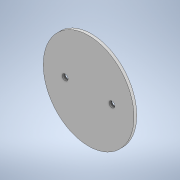
# Autodesk Inventor part: Plato da Valvula
Saved by Autodesk Inventor 2022 (Build 260153000, 153)
## iProperties
Created: 2022-06-22
Part Number: Plato da Valvula
Material: Genérico
Document SubType Name: Modeling
Designer: robofei
Density: 1 g/cm^3
Appearance: Padrão
Author: robofei
Autodesk Inventor part; units mm, degrees
ref_plane "YZ Plane" through (0, 0, 0) normal (1, 0, 0) x (0, 1, 0)
ref_plane "XZ Plane" through (0, 0, 0) normal (0, 1, 0) x (-1, 0, 0)
ref_plane "XY Plane" through (0, 0, 0) normal (0, 0, 1) x (1, 0, 0)
sketch "Esboço1" plane through (0, 0, 0) normal (0, 0, 1) x (1, 0, 0)
  ellipse E0 centre (0, 0) end of major axis (96.9, 0) minor radius 102.5
  circle A0 centre (-50, 0) radius 6.25
  circle A1 centre (50, 0) radius 6.25
  dimension "d0" = 96.9
  dimension "d1" = 102.5
  dimension "d2" = 100
  dimension "d3" = 50
  dimension "d4" = 12.5
  dimension "d5" = 12.5
  constraints: 3 centre point, 1 coincident, 1 other
  measures "d2" distance of A1.centre A0.centre
  measures "d3" distance of point (0, 0) A0.centre
  measures "d4" diameter of A0
  measures "d5" diameter of A1
extrude "Extrusão1" add sketch "Esboço1" along normal blind 6
